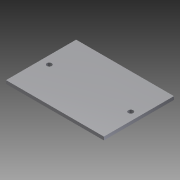
# Autodesk Inventor part: cetakan sepatu 1
Saved by Autodesk Inventor 2012 (Build 160160000, 160)
## iProperties
Created: 2014-01-20
Part Number: cetakan sepatu 1
Material: Default
Document SubType Name: Modeling
Designer: Irwan Haryanto
Density: 1 g/cm^3
Author: Irwan Haryanto
Autodesk Inventor part; units mm, degrees
ref_plane "YZ Plane" through (0, 0, 0) normal (1, 0, 0) x (0, 1, 0)
ref_plane "XZ Plane" through (0, 0, 0) normal (0, 1, 0) x (-1, 0, 0)
ref_plane "XY Plane" through (0, 0, 0) normal (0, 0, 1) x (1, 0, 0)
sketch "Sketch1" plane through (0, 0, 0) normal (0, 0, 1) x (1, 0, 0)
  line L0 (-190.4003, -106.9233) -> (-190.4003, -63.9233)
  line L1 (-190.4003, -63.9233) -> (-250.4003, -63.9233)
  line L2 (-250.4003, -63.9233) -> (-250.4003, -106.9233)
  line L3 (-250.4003, -106.9233) -> (-190.4003, -106.9233)
  circle A0 centre (-245.4003, -85.4233) radius 1.5
  circle A1 centre (-195.4003, -85.4233) radius 1.5
  point P0 (0, 0)
  dimension "d0" = 60
  dimension "d1" = 43
  dimension "d2" = 3
  dimension "d3" = 21.5
  dimension "d4" = 5
  dimension "d5" = 3
  dimension "d6" = 5
  dimension "d7" = 21.5
  constraints: 8 end point, 2 centre point, 2 perpendicular
  measures "d0" distance of L0.end L2.start
  measures "d1" distance of L2.start L2.end
  measures "d2" diameter of A0
  measures "d3" distance from line of A0.centre L1
  measures "d4" distance from line of L2 A0.centre
  measures "d5" diameter of A1
  measures "d6" distance from line of L0 A1.centre
  measures "d7" distance from line of A1.centre L1
extrude "Extrusion1" add sketch "Sketch1" along normal blind 2
body "Solid1"
